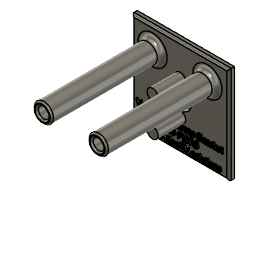
Vekooto Antenna Bracket v1.3 (Autodesk Fusion 360 design; units mm, degrees)
part number: 2026-07-18-22-31-47-243
Autodesk Fusion 360 part; units mm, degrees
note: some values were not read from the file. Chosen so that the rebuilt part matches the saved one: which face or edge a step refers to; the layout of a text; which pieces of a blend or face edit are solid.
(part 1 of 2)
sketch "Sketch1" plane through (0, 0, 0) normal (0, 0, 1) x (1, 0, 0)
  line L0 (22.352, -22.352) -> (-22.352, -22.352)
  line L1 (-22.352, -22.352) -> (-22.352, 22.352)
  line L2 (-22.352, 22.352) -> (22.352, 22.352)
  line L3 (22.352, 22.352) -> (22.352, -22.352)
  line L4 (22.352, -22.352) -> (-22.352, 22.352) construction
  line L5 (-22.352, -22.352) -> (22.352, 22.352) construction
  dimension "d4" = 44.704
  dimension "d5" = 44.704
  constraint horizontal L0
  constraint perpendicular L0 L1
  constraint parallel L0 L2
  constraint parallel L1 L3
  constraint coincident L4 origin
  constraint coincident L5 origin
  measures "d4" distance of L1.end L2.end
  measures "d5" distance of L0.end L1.end
extrude "Extrude1" add sketch "Sketch1" along normal blind 2.54
sketch "Sketch2" plane through (0, 0, 2.54) normal (0, 0, 1) x (1, 0, 0)
  line L0 (22.352, 22.352) -> (-22.352, 22.352)
  line L1 (-22.352, 22.352) -> (-22.352, -22.352)
  line L2 (-22.352, -22.352) -> (22.352, -22.352)
  line L3 (22.352, -22.352) -> (22.352, 22.352)
  circle A0 centre (0, 0) radius 5.08
  dimension "d8" = 10.16
  constraint coincident A0.centre origin
  measures "d8" diameter of A0
extrude "Extrude2" cut sketch "Sketch2" against normal blind 2.54 contours A0
sketch "Sketch3" plane through (0, 0, 2.54) normal (0, 0, 1) x (1, 0, 0)
  circle A0 centre (0, 0) radius 5.08
  line L0 (22.352, 22.352) -> (-22.352, 22.352)
  line L1 (-22.352, 22.352) -> (-22.352, -22.352)
  line L2 (-22.352, -22.352) -> (22.352, -22.352)
  line L3 (22.352, -22.352) -> (22.352, 22.352)
  circle A1 centre (-15.8649, 0) radius 4.445
  dimension "d13" = 8.89
  measures "d13" diameter of A1
extrude "Extrude3" add sketch "Sketch3" along normal blind 50.8 contours A1
move_face "MoveFace1" to x (1, 0, 0) y (0, 1, 0) z (0, 0, 1) at (2.54, 0, 0) 1 faces at (-11.442, -0.4426, 36.4067)
move_face "MoveFace2" to x (1, 0, 0) y (0, 1, 0) z (0, 0, 1) at (2.54, 12.7, 0) 2 faces at (-8.902, 0.4426, 36.4067) (-13.1059, 0.033, 53.34)
sketch "Sketch4" plane through (0, 0, 2.54) normal (0, 0, 1) x (1, 0, 0)
  circle A0 centre (-10.7849, 12.7) radius 4.445
  circle A1 centre (0, 0) radius 5.08
  line L0 (22.352, 22.352) -> (-22.352, 22.352)
  line L1 (-22.352, 22.352) -> (-22.352, -22.352)
  line L2 (-22.352, -22.352) -> (22.352, -22.352)
  line L3 (22.352, -22.352) -> (22.352, 22.352)
  circle A2 centre (11.9328, 13.2113) radius 4.445
  dimension "d18" = 8.89
  measures "d18" diameter of A2
extrude "Extrude4" add sketch "Sketch4" along normal blind 50.8 contours A2
move_face "MoveFace3" to x (1, 0, 0) y (0, 1, 0) z (0, 0, 1) at (0, -0.508, 0) 1 faces at (16.3557, 12.7687, 36.4067)
move_face "MoveFace4" to x (1, 0, 0) y (0, 1, 0) z (0, 0, 1) at (-2.54, 0, 0) 1 faces at (-6.362, 13.1426, 36.4067)
move_face "MoveFace5" to x (1, 0, 0) y (0, 1, 0) z (0, 0, 1) at (0.508, 0, 0) 1 faces at (16.3557, 13.1458, 36.4067)
move_face "MoveFace6" to x (1, 0, 0) y (0, 1, 0) z (0, 0, 1) at (0.508, 0, 0) 1 faces at (-8.902, 13.1426, 36.4067)
sketch "Sketch5" plane through (0, 0, 53.34) normal (0, 0, 1) x (1, 0, 0)
  circle A0 centre (-12.8169, 12.7) radius 4.445
  circle A1 centre (-12.8169, 12.7) radius 2.54
  dimension "d22" = 5.08
  constraint concentric A0 A1
  measures "d22" diameter of A1
sketch "Sketch6" plane through (0, 0, 53.34) normal (0, 0, 1) x (1, 0, 0)
  circle A0 centre (12.4408, 12.7033) radius 4.445
  circle A1 centre (12.4408, 12.7033) radius 2.54
  dimension "d23" = 5.08
  constraint concentric A0 A1
  measures "d23" diameter of A1
extrude "Extrude5" cut sketch "Sketch5" against normal blind 50.8 contours A1
extrude "Extrude6" cut sketch "Sketch6" against normal blind 50.8 contours A1
fillet "Fillet1" radius 2.286 1 edges at (8.2966, 14.3106, 2.54)
fillet "Fillet2" radius 2.286 1 edges at (-16.9611, 14.3074, 2.54)
fillet "Fillet3" radius 0.762 4 edges at (-15.185, 13.6185, 53.34) (-16.9611, 11.0926, 53.34) (10.0726, 13.6218, 53.34) (8.2966, 11.0959, 53.34)
fillet "Fillet4" radius 1.016 4 edges at (0, -22.352, 2.54) (-22.352, 0, 2.54) (0, 22.352, 2.54) (22.352, 0, 2.54)
sketch "Sketch7" plane through (0, 0, 0) normal (0, 0, -1) x (-1, 0, 0)
  circle A0 centre (0, 0) radius 5.08
  line L0 (22.352, 22.352) -> (-22.352, 22.352)
  line L1 (-22.352, 22.352) -> (-22.352, -22.352)
  line L2 (-22.352, -22.352) -> (22.352, -22.352)
  line L3 (22.352, -22.352) -> (22.352, 22.352)
  line L4 (-22.3513, 12.9981) -> (22.3527, 13.0094) construction
  line L5 (22.3527, 13.0094) -> (22.3513, 18.5497) construction
  line L6 (22.3513, 18.5497) -> (-22.3527, 18.5384) construction
  line L7 (-22.3527, 18.5384) -> (-22.3513, 12.9981) construction
  dimension "d36" = 2.54
  dimension "d37" = 0
  text T0 "Vekooto Antenna Bracket v.1.1" font "Arial" height 2.54 align centre top in box 44.704 x 5.5403 at (-22.3513, 12.9981) x (1, 0.000252) y (-0.000252, 1) spacing 1 kerned
  constraint coincident L3
  constraint coincident L1
extrude "Extrude7" cut sketch "Sketch7" against normal blind 0.762 text T0
sketch "Sketch8" plane through (0, 0, 0) normal (0, 0, -1) x (-1, 0, 0)
  line L0 (22.352, 22.352) -> (-22.352, 22.352)
  line L1 (-22.352, 22.352) -> (-22.352, -22.352)
  line L2 (-22.352, -22.352) -> (22.352, -22.352)
  line L3 (22.352, -22.352) -> (22.352, 22.352)
  circle A0 centre (0, 0) radius 5.08
  line L4 (-17.5814, 18.5396) -> (-18.5753, 15.9994)
  line L5 (-18.5753, 15.9994) -> (-18.9201, 15.9993)
  line L6 (-18.9201, 15.9993) -> (-19.9049, 18.5391)
  line L7 (-19.9049, 18.5391) -> (-19.541, 18.5391)
  line L8 (-19.541, 18.5391) -> (-18.8804, 16.6941)
  spline S0 degree 3 poles (-18.8804, 16.6941) (-18.8553, 16.6227) (-18.807, 16.4853) (-18.7664, 16.3455) (-18.7469, 16.2783) knots 0 0 0 0 0.022697 0.043678 0.043678 0.043678 0.043678
  spline S1 degree 3 poles (-18.7469, 16.2783) (-18.7264, 16.3478) (-18.6851, 16.4879) (-18.6353, 16.6251) (-18.6102, 16.6942) knots 0 0 0 0 0.021744 0.043787 0.043787 0.043787 0.043787
  line L9 (-18.6102, 16.6942) -> (-17.9245, 18.5395)
  line L10 (-17.9245, 18.5395) -> (-17.5814, 18.5396)
  line L11 (-15.2281, 16.7297) -> (-15.2279, 16.0002)
  line L12 (-15.2279, 16.0002) -> (-15.5398, 16.0001)
  line L13 (-15.5398, 16.0001) -> (-15.5404, 18.5401)
  line L14 (-15.5404, 18.5401) -> (-15.2286, 18.5402)
  line L15 (-15.2286, 18.5402) -> (-15.2282, 17.0918)
  line L16 (-15.2282, 17.0918) -> (-14.4903, 17.8404)
  line L17 (-14.4903, 17.8404) -> (-14.0866, 17.8405)
  line L18 (-14.0866, 17.8405) -> (-14.7899, 17.1577)
  line L19 (-14.7899, 17.1577) -> (-14.0151, 16.0005)
  line L20 (-14.0151, 16.0005) -> (-14.3997, 16.0004)
  line L21 (-14.3997, 16.0004) -> (-15.0081, 16.9411)
  line L22 (-15.0081, 16.9411) -> (-15.2281, 16.7297)
  spline S2 degree 3 poles (-11.0471, 15.9597) (-11.1683, 15.9686) (-11.403, 15.9857) (-11.5842, 16.1351) (-11.6718, 16.2073) knots 0 0 0 0 0.035478 0.06869 0.06869 0.06869 0.06869
  spline S3 degree 3 poles (-11.6718, 16.2073) (-11.7412, 16.3046) (-11.8927, 16.5171) (-11.9041, 16.7791) (-11.9102, 16.9211) knots 0 0 0 0 0.035119 0.076697 0.076697 0.076697 0.076697
  spline S4 degree 3 poles (-11.9102, 16.9211) (-11.9032, 17.076) (-11.8902, 17.3608) (-11.709, 17.5788) (-11.6263, 17.6783) knots 0 0 0 0 0.045048 0.082857 0.082857 0.082857 0.082857
  spline S5 degree 3 poles (-11.6263, 17.6783) (-11.5415, 17.7379) (-11.368, 17.8601) (-11.1561, 17.8752) (-11.0476, 17.8829) knots 0 0 0 0 0.030474 0.062419 0.062419 0.062419 0.062419
  spline S6 degree 3 poles (-11.0476, 17.8829) (-10.928, 17.8737) (-10.6948, 17.8557) (-10.5149, 17.7069) (-10.4273, 17.6344) knots 0 0 0 0 0.035035 0.068301 0.068301 0.068301 0.068301
  spline S7 degree 3 poles (-10.4273, 17.6344) (-10.3571, 17.5394) (-10.2069, 17.336) (-10.1934, 17.0825) (-10.1863, 16.9475) knots 0 0 0 0 0.034681 0.074234 0.074234 0.074234 0.074234
  spline S8 degree 3 poles (-10.1863, 16.9475) (-10.1883, 16.8403) (-10.192, 16.6476) (-10.2617, 16.4683) (-10.2927, 16.3887) knots 0 0 0 0 0.03184 0.057276 0.057276 0.057276 0.057276
  spline S9 degree 3 poles (-10.2927, 16.3887) (-10.3324, 16.3246) (-10.4119, 16.1959) (-10.539, 16.1137) (-10.6028, 16.0724) knots 0 0 0 0 0.022319 0.044787 0.044787 0.044787 0.044787
  spline S10 degree 3 poles (-10.6028, 16.0724) (-10.6725, 16.0396) (-10.8133, 15.9732) (-10.9687, 15.9642) (-11.0471, 15.9597) knots 0 0 0 0 0.022904 0.046226 0.046226 0.046226 0.046226
  spline S11 degree 3 poles (-8.0879, 15.9604) (-8.2091, 15.9693) (-8.4437, 15.9865) (-8.6249, 16.1358) (-8.7125, 16.208) knots 0 0 0 0 0.035479 0.06869 0.06869 0.06869 0.06869
  spline S12 degree 3 poles (-8.7125, 16.208) (-8.7819, 16.3054) (-8.9334, 16.5179) (-8.9448, 16.7798) (-8.9509, 16.9218) knots 0 0 0 0 0.035119 0.076697 0.076697 0.076697 0.076697
  spline S13 degree 3 poles (-8.9509, 16.9218) (-8.9439, 17.0767) (-8.9309, 17.3616) (-8.7497, 17.5796) (-8.667, 17.679) knots 0 0 0 0 0.045048 0.082857 0.082857 0.082857 0.082857
  spline S14 degree 3 poles (-8.667, 17.679) (-8.5823, 17.7387) (-8.4087, 17.8608) (-8.1968, 17.8759) (-8.0883, 17.8836) knots 0 0 0 0 0.030474 0.062419 0.062419 0.062419 0.062419
  spline S15 degree 3 poles (-8.0883, 17.8836) (-7.9687, 17.8744) (-7.7356, 17.8565) (-7.5556, 17.7076) (-7.468, 17.6352) knots 0 0 0 0 0.035035 0.068301 0.068301 0.068301 0.068301
  spline S16 degree 3 poles (-7.468, 17.6352) (-7.3978, 17.5401) (-7.2476, 17.3367) (-7.2342, 17.0833) (-7.227, 16.9482) knots 0 0 0 0 0.034681 0.074234 0.074234 0.074234 0.074234
  spline S17 degree 3 poles (-7.227, 16.9482) (-7.229, 16.8411) (-7.2327, 16.6483) (-7.3025, 16.4691) (-7.3334, 16.3895) knots 0 0 0 0 0.03184 0.057276 0.057276 0.057276 0.057276
  spline S18 degree 3 poles (-7.3334, 16.3895) (-7.3731, 16.3253) (-7.4526, 16.1966) (-7.5797, 16.1144) (-7.6435, 16.0732) knots 0 0 0 0 0.022319 0.044787 0.044787 0.044787 0.044787
  spline S19 degree 3 poles (-7.6435, 16.0732) (-7.7132, 16.0403) (-7.854, 15.974) (-8.0094, 15.965) (-8.0879, 15.9604) knots 0 0 0 0 0.022904 0.046226 0.046226 0.046226 0.046226
  line L23 (-3.3928, 17.0081) -> (-3.3925, 16.0032)
  line L24 (-3.3925, 16.0032) -> (-3.7044, 16.0031)
  line L25 (-3.7044, 16.0031) -> (-3.7048, 17.8432)
  line L26 (-3.7048, 17.8432) -> (-3.4242, 17.8432)
  line L27 (-3.4242, 17.8432) -> (-3.4241, 17.5816)
  spline S20 degree 3 poles (-3.4241, 17.5816) (-3.3481, 17.67) (-3.1939, 17.8496) (-2.9582, 17.873) (-2.8385, 17.885) knots 0 0 0 0 0.03363 0.068256 0.068256 0.068256 0.068256
  spline S21 degree 3 poles (-2.8385, 17.885) (-2.7848, 17.8827) (-2.6798, 17.8784) (-2.581, 17.8427) (-2.5327, 17.8253) knots 0 0 0 0 0.016031 0.031322 0.031322 0.031322 0.031322
  spline S22 degree 3 poles (-2.5327, 17.8253) (-2.49, 17.8049) (-2.4097, 17.7667) (-2.3513, 17.6998) (-2.3239, 17.6685) knots 0 0 0 0 0.014014 0.026358 0.026358 0.026358 0.026358
  spline S23 degree 3 poles (-2.3239, 17.6685) (-2.3024, 17.6339) (-2.2578, 17.5623) (-2.2374, 17.4804) (-2.2268, 17.4381) knots 0 0 0 0 0.012138 0.02514 0.02514 0.02514 0.02514
  spline S24 degree 3 poles (-2.2268, 17.4381) (-2.2218, 17.3984) (-2.2091, 17.2978) (-2.2093, 17.1964) (-2.2094, 17.1349) knots 0 0 0 0 0.011982 0.030396 0.030396 0.030396 0.030396
  line L28 (-2.2094, 17.1349) -> (-2.2091, 16.0035)
  line L29 (-2.2091, 16.0035) -> (-2.521, 16.0034)
  line L30 (-2.521, 16.0034) -> (-2.5213, 17.1227)
  spline S25 degree 3 poles (-2.5213, 17.1227) (-2.5216, 17.1786) (-2.5221, 17.2752) (-2.5472, 17.3684) (-2.5577, 17.4077) knots 0 0 0 0 0.016679 0.028836 0.028836 0.028836 0.028836
  spline S26 degree 3 poles (-2.5577, 17.4077) (-2.5725, 17.4377) (-2.6026, 17.499) (-2.6584, 17.5384) (-2.6869, 17.5584) knots 0 0 0 0 0.009876 0.020131 0.020131 0.020131 0.020131
  spline S27 degree 3 poles (-2.6869, 17.5584) (-2.7198, 17.5748) (-2.7882, 17.6089) (-2.8647, 17.6127) (-2.9043, 17.6147) knots 0 0 0 0 0.01092 0.022678 0.022678 0.022678 0.022678
  spline S28 degree 3 poles (-2.9043, 17.6147) (-2.9682, 17.6096) (-3.0947, 17.5995) (-3.1974, 17.525) (-3.2482, 17.4881) knots 0 0 0 0 0.018828 0.037284 0.037284 0.037284 0.037284
  spline S29 degree 3 poles (-3.2482, 17.4881) (-3.2901, 17.429) (-3.3908, 17.2868) (-3.392, 17.1109) (-3.3928, 17.0081) knots 0 0 0 0 0.021294 0.051185 0.051185 0.051185 0.051185
  spline S30 degree 3 poles (0.0293, 16.2189) (0.0837, 16.2221) (0.1888, 16.2284) (0.2787, 16.2828) (0.3221, 16.3091) knots 0 0 0 0 0.016056 0.031049 0.031049 0.031049 0.031049
  spline S31 degree 3 poles (0.3221, 16.3091) (0.3613, 16.3461) (0.4471, 16.427) (0.4907, 16.537) (0.5144, 16.5967) knots 0 0 0 0 0.015968 0.034972 0.034972 0.034972 0.034972
  line L31 (0.5144, 16.5967) -> (0.8366, 16.557)
  spline S32 degree 3 poles (0.8366, 16.557) (0.8071, 16.469) (0.7498, 16.2989) (0.618, 16.1773) (0.5543, 16.1185) knots 0 0 0 0 0.027335 0.052897 0.052897 0.052897 0.052897
  spline S33 degree 3 poles (0.5543, 16.1185) (0.4781, 16.0731) (0.3162, 15.9766) (0.1275, 15.9674) (0.0277, 15.9625) knots 0 0 0 0 0.026229 0.055682 0.055682 0.055682 0.055682
  spline S34 degree 3 poles (0.0277, 15.9625) (-0.0979, 15.9708) (-0.3381, 15.9866) (-0.5239, 16.1385) (-0.6126, 16.2109) knots 0 0 0 0 0.03672 0.070219 0.070219 0.070219 0.070219
  spline S35 degree 3 poles (-0.6126, 16.2109) (-0.6815, 16.307) (-0.8303, 16.5146) (-0.8427, 16.7707) (-0.8493, 16.9083) knots 0 0 0 0 0.034736 0.075044 0.075044 0.075044 0.075044
  spline S36 degree 3 poles (-0.8493, 16.9083) (-0.8428, 17.0504) (-0.8308, 17.3142) (-0.6799, 17.5297) (-0.6103, 17.6291) knots 0 0 0 0 0.041667 0.077342 0.077342 0.077342 0.077342
  spline S37 degree 3 poles (-0.6103, 17.6291) (-0.5233, 17.7039) (-0.345, 17.8571) (-0.1103, 17.876) (0.0099, 17.8857) knots 0 0 0 0 0.033526 0.068681 0.068681 0.068681 0.068681
  spline S38 degree 3 poles (0.0099, 17.8857) (0.1264, 17.8761) (0.3548, 17.8574) (0.528, 17.7078) (0.6129, 17.6346) knots 0 0 0 0 0.034109 0.066844 0.066844 0.066844 0.066844
  spline S39 degree 3 poles (0.6129, 17.6346) (0.681, 17.5372) (0.8288, 17.3259) (0.8406, 17.0672) (0.847, 16.9277) knots 0 0 0 0 0.034955 0.075831 0.075831 0.075831 0.075831
  spline S40 degree 3 poles (0.847, 16.9277) (0.8468, 16.9162) (0.8466, 16.8885) (0.8457, 16.8608) (0.8452, 16.8446) knots 0 0 0 0 0.003465 0.008319 0.008319 0.008319 0.008319
  line L32 (0.8452, 16.8446) -> (-0.527, 16.8442)
  spline S41 degree 3 poles (-0.527, 16.8442) (-0.5179, 16.7519) (-0.5013, 16.5814) (-0.4012, 16.4432) (-0.3553, 16.3799) knots 0 0 0 0 0.02726 0.050297 0.050297 0.050297 0.050297
  spline S42 degree 3 poles (-0.3553, 16.3799) (-0.3004, 16.333) (-0.1895, 16.2381) (-0.0441, 16.2254) (0.0293, 16.2189) knots 0 0 0 0 0.021124 0.042642 0.042642 0.042642 0.042642
  line L33 (3.5134, 17.0099) -> (3.5137, 16.0049)
  line L34 (3.5137, 16.0049) -> (3.2018, 16.0049)
  line L35 (3.2018, 16.0049) -> (3.2013, 17.8449)
  line L36 (3.2013, 17.8449) -> (3.482, 17.845)
  line L37 (3.482, 17.845) -> (3.4821, 17.5833)
  spline S43 degree 3 poles (3.4821, 17.5833) (3.558, 17.6718) (3.7122, 17.8513) (3.948, 17.8748) (4.0676, 17.8867) knots 0 0 0 0 0.03363 0.068256 0.068256 0.068256 0.068256
  spline S44 degree 3 poles (4.0676, 17.8867) (4.1214, 17.8845) (4.2264, 17.8801) (4.3252, 17.8444) (4.3734, 17.827) knots 0 0 0 0 0.016031 0.031322 0.031322 0.031322 0.031322
  spline S45 degree 3 poles (4.3734, 17.827) (4.4162, 17.8067) (4.4965, 17.7685) (4.5549, 17.7016) (4.5823, 17.6702) knots 0 0 0 0 0.014014 0.026358 0.026358 0.026358 0.026358
  spline S46 degree 3 poles (4.5823, 17.6702) (4.6038, 17.6357) (4.6484, 17.5641) (4.6688, 17.4822) (4.6793, 17.4398) knots 0 0 0 0 0.012138 0.02514 0.02514 0.02514 0.02514
  spline S47 degree 3 poles (4.6793, 17.4398) (4.6844, 17.4002) (4.6971, 17.2996) (4.6969, 17.1981) (4.6968, 17.1366) knots 0 0 0 0 0.011982 0.030396 0.030396 0.030396 0.030396
  line L38 (4.6968, 17.1366) -> (4.697, 16.0052)
  line L39 (4.697, 16.0052) -> (4.3852, 16.0052)
  line L40 (4.3852, 16.0052) -> (4.3849, 17.1244)
  spline S48 degree 3 poles (4.3849, 17.1244) (4.3846, 17.1803) (4.384, 17.277) (4.359, 17.3701) (4.3484, 17.4094) knots 0 0 0 0 0.016679 0.028836 0.028836 0.028836 0.028836
  spline S49 degree 3 poles (4.3484, 17.4094) (4.3337, 17.4395) (4.3036, 17.5007) (4.2478, 17.5401) (4.2193, 17.5601) knots 0 0 0 0 0.009876 0.02013 0.02013 0.02013 0.02013
  spline S50 degree 3 poles (4.2193, 17.5601) (4.1864, 17.5765) (4.1179, 17.6106) (4.0415, 17.6144) (4.0019, 17.6164) knots 0 0 0 0 0.01092 0.022678 0.022678 0.022678 0.022678
  spline S51 degree 3 poles (4.0019, 17.6164) (3.938, 17.6113) (3.8114, 17.6013) (3.7088, 17.5267) (3.658, 17.4898) knots 0 0 0 0 0.018828 0.037284 0.037284 0.037284 0.037284
  spline S52 degree 3 poles (3.658, 17.4898) (3.6161, 17.4307) (3.5154, 17.2886) (3.5141, 17.1126) (3.5134, 17.0099) knots 0 0 0 0 0.021294 0.051185 0.051185 0.051185 0.051185
  line L41 (6.764, 16.0058) -> (6.4383, 16.0057)
  spline S53 degree 3 poles (6.4383, 16.0057) (6.4235, 16.0403) (6.3923, 16.1131) (6.3815, 16.1915) (6.3759, 16.2326) knots 0 0 0 0 0.011255 0.023633 0.023633 0.023633 0.023633
  spline S54 degree 3 poles (6.3759, 16.2326) (6.3209, 16.188) (6.2183, 16.1048) (6.0982, 16.05) (6.0424, 16.0246) knots 0 0 0 0 0.021138 0.039444 0.039444 0.039444 0.039444
  spline S55 degree 3 poles (6.0424, 16.0246) (5.9875, 16.0069) (5.8757, 15.9709) (5.7582, 15.9663) (5.6985, 15.9639) knots 0 0 0 0 0.017222 0.035068 0.035068 0.035068 0.035068
  spline S56 degree 3 poles (5.6985, 15.9639) (5.6062, 15.9676) (5.4365, 15.9743) (5.2963, 16.0688) (5.2324, 16.1119) knots 0 0 0 0 0.027067 0.049766 0.049766 0.049766 0.049766
  spline S57 degree 3 poles (5.2324, 16.1119) (5.1849, 16.1652) (5.0886, 16.2732) (5.0759, 16.4174) (5.0694, 16.4905) knots 0 0 0 0 0.020829 0.042207 0.042207 0.042207 0.042207
  spline S58 degree 3 poles (5.0694, 16.4905) (5.0718, 16.5342) (5.0765, 16.6205) (5.1129, 16.6988) (5.1309, 16.7374) knots 0 0 0 0 0.013021 0.025653 0.025653 0.025653 0.025653
  spline S59 degree 3 poles (5.1309, 16.7374) (5.1527, 16.7726) (5.1957, 16.842) (5.2602, 16.8921) (5.292, 16.9167) knots 0 0 0 0 0.012324 0.024281 0.024281 0.024281 0.024281
  spline S60 degree 3 poles (5.292, 16.9167) (5.3266, 16.938) (5.3971, 16.9813) (5.4761, 17.0063) (5.5163, 17.019) knots 0 0 0 0 0.01214 0.024739 0.024739 0.024739 0.024739
  spline S61 degree 3 poles (5.5163, 17.019) (5.5546, 17.0275) (5.6462, 17.0477) (5.7393, 17.0592) (5.7935, 17.0659) knots 0 0 0 0 0.011766 0.028127 0.028127 0.028127 0.028127
  spline S62 degree 3 poles (5.7935, 17.0659) (5.9034, 17.0792) (6.0915, 17.102) (6.2739, 17.1525) (6.3496, 17.1734) knots 0 0 0 0 0.033159 0.056713 0.056713 0.056713 0.056713
  spline S63 degree 3 poles (6.3496, 17.1734) (6.3501, 17.1909) (6.3509, 17.218) (6.3512, 17.2452) (6.3514, 17.2549) knots 0 0 0 0 0.005243 0.008145 0.008145 0.008145 0.008145
  spline S64 degree 3 poles (6.3514, 17.2549) (6.3501, 17.3112) (6.3479, 17.4106) (6.2886, 17.4893) (6.2629, 17.5234) knots 0 0 0 0 0.016393 0.028904 0.028904 0.028904 0.028904
  spline S65 degree 3 poles (6.2629, 17.5234) (6.2148, 17.5541) (6.107, 17.6228) (5.9787, 17.6268) (5.9077, 17.629) knots 0 0 0 0 0.016839 0.037669 0.037669 0.037669 0.037669
  spline S66 degree 3 poles (5.9077, 17.629) (5.8426, 17.628) (5.7281, 17.6262) (5.6266, 17.5742) (5.5829, 17.5518) knots 0 0 0 0 0.01922 0.03378 0.03378 0.03378 0.03378
  spline S67 degree 3 poles (5.5829, 17.5518) (5.5495, 17.518) (5.4738, 17.4413) (5.4443, 17.3371) (5.4279, 17.2789) knots 0 0 0 0 0.014041 0.031838 0.031838 0.031838 0.031838
  line L42 (5.4279, 17.2789) -> (5.1229, 17.3204)
  spline S68 degree 3 poles (5.1229, 17.3204) (5.1378, 17.3809) (5.1656, 17.4942) (5.2298, 17.5914) (5.2597, 17.6366) knots 0 0 0 0 0.01853 0.034684 0.034684 0.034684 0.034684
  spline S69 degree 3 poles (5.2597, 17.6366) (5.2966, 17.675) (5.3749, 17.7565) (5.4797, 17.7994) (5.5352, 17.8221) knots 0 0 0 0 0.01579 0.033533 0.033533 0.033533 0.033533
  spline S70 degree 3 poles (5.5352, 17.8221) (5.5995, 17.841) (5.7358, 17.8811) (5.8778, 17.8851) (5.9527, 17.8872) knots 0 0 0 0 0.02005 0.042416 0.042416 0.042416 0.042416
  spline S71 degree 3 poles (5.9527, 17.8872) (6.0244, 17.886) (6.1546, 17.8838) (6.2795, 17.8479) (6.3356, 17.8318) knots 0 0 0 0 0.021399 0.038838 0.038838 0.038838 0.038838
  spline S72 degree 3 poles (6.3356, 17.8318) (6.3801, 17.8138) (6.4612, 17.7808) (6.5239, 17.7199) (6.5522, 17.6924) knots 0 0 0 0 0.014228 0.025974 0.025974 0.025974 0.025974
  spline S73 degree 3 poles (6.5522, 17.6924) (6.5738, 17.6616) (6.6191, 17.5969) (6.6389, 17.5203) (6.6493, 17.4802) knots 0 0 0 0 0.011185 0.023506 0.023506 0.023506 0.023506
  spline S74 degree 3 poles (6.6493, 17.4802) (6.6538, 17.443) (6.6654, 17.3475) (6.6651, 17.2513) (6.665, 17.1926) knots 0 0 0 0 0.011236 0.028827 0.028827 0.028827 0.028827
  line L43 (6.665, 17.1926) -> (6.6651, 16.7767)
  spline S75 degree 3 poles (6.6651, 16.7767) (6.6644, 16.6583) (6.6633, 16.4746) (6.6794, 16.2917) (6.6851, 16.2266) knots 0 0 0 0 0.0355 0.055071 0.055071 0.055071 0.055071
  spline S76 degree 3 poles (6.6851, 16.2266) (6.6935, 16.1885) (6.7104, 16.1115) (6.746, 16.0412) (6.764, 16.0058) knots 0 0 0 0 0.011667 0.02354 0.02354 0.02354 0.02354
  line L44 (10.8094, 16.9701) -> (10.8097, 16.0068)
  line L45 (10.8097, 16.0068) -> (10.4978, 16.0067)
  line L46 (10.4978, 16.0067) -> (10.4973, 17.8467)
  line L47 (10.4973, 17.8467) -> (10.778, 17.8468)
  line L48 (10.778, 17.8468) -> (10.7781, 17.5678)
  spline S77 degree 3 poles (10.7781, 17.5678) (10.8093, 17.6245) (10.8625, 17.7209) (10.9432, 17.7954) (10.9764, 17.8261) knots 0 0 0 0 0.01925 0.032742 0.032742 0.032742 0.032742
  spline S78 degree 3 poles (10.9764, 17.8261) (11.0074, 17.8443) (11.0693, 17.8806) (11.1408, 17.8858) (11.1765, 17.8885) knots 0 0 0 0 0.010635 0.021211 0.021211 0.021211 0.021211
  spline S79 degree 3 poles (11.1765, 17.8885) (11.2305, 17.8835) (11.3444, 17.873) (11.4445, 17.8173) (11.4971, 17.7881) knots 0 0 0 0 0.016094 0.033922 0.033922 0.033922 0.033922
  line L49 (11.4971, 17.7881) -> (11.3897, 17.4987)
  spline S80 degree 3 poles (11.3897, 17.4987) (11.3524, 17.5184) (11.2806, 17.5563) (11.1998, 17.563) (11.161, 17.5662) knots 0 0 0 0 0.012508 0.024067 0.024067 0.024067 0.024067
  spline S81 degree 3 poles (11.161, 17.5662) (11.1278, 17.5636) (11.0614, 17.5585) (11.0054, 17.5226) (10.9774, 17.5047) knots 0 0 0 0 0.009824 0.019638 0.019638 0.019638 0.019638
  spline S82 degree 3 poles (10.9774, 17.5047) (10.952, 17.4816) (10.8997, 17.4341) (10.8744, 17.368) (10.8613, 17.334) knots 0 0 0 0 0.010126 0.020898 0.020898 0.020898 0.020898
  spline S83 degree 3 poles (10.8613, 17.334) (10.8462, 17.2762) (10.8149, 17.157) (10.8113, 17.0337) (10.8094, 16.9701) knots 0 0 0 0 0.017844 0.03686 0.03686 0.03686 0.03686
  spline S84 degree 3 poles (14.3944, 16.2225) (14.4525, 16.2267) (14.5657, 16.2349) (14.6567, 16.3024) (14.701, 16.3352) knots 0 0 0 0 0.017083 0.033278 0.033278 0.033278 0.033278
  spline S85 degree 3 poles (14.701, 16.3352) (14.7386, 16.3809) (14.8216, 16.4819) (14.8444, 16.6111) (14.8569, 16.6818) knots 0 0 0 0 0.017473 0.038572 0.038572 0.038572 0.038572
  line L50 (14.8569, 16.6818) -> (15.1635, 16.642)
  spline S86 degree 3 poles (15.1635, 16.642) (15.1419, 16.5435) (15.1004, 16.3546) (14.9692, 16.2132) (14.9064, 16.1455) knots 0 0 0 0 0.029645 0.056823 0.056823 0.056823 0.056823
  spline S87 degree 3 poles (14.9064, 16.1455) (14.8322, 16.0932) (14.6798, 15.9858) (14.4935, 15.9728) (14.3979, 15.9661) knots 0 0 0 0 0.0267 0.054846 0.054846 0.054846 0.054846
  spline S88 degree 3 poles (14.3979, 15.9661) (14.2795, 15.975) (14.0501, 15.9921) (13.8752, 16.1409) (13.7906, 16.2128) knots 0 0 0 0 0.034622 0.067083 0.067083 0.067083 0.067083
  spline S89 degree 3 poles (13.7906, 16.2128) (13.7237, 16.3097) (13.5774, 16.5217) (13.5667, 16.7802) (13.5608, 16.9206) knots 0 0 0 0 0.034624 0.075764 0.075764 0.075764 0.075764
  spline S90 degree 3 poles (13.5608, 16.9206) (13.564, 17.0147) (13.5701, 17.1937) (13.6307, 17.3622) (13.6594, 17.4421) knots 0 0 0 0 0.028047 0.053368 0.053368 0.053368 0.053368
  spline S91 degree 3 poles (13.6594, 17.4421) (13.6961, 17.5116) (13.7683, 17.6486) (13.8967, 17.7349) (13.96, 17.7774) knots 0 0 0 0 0.023185 0.045661 0.045661 0.045661 0.045661
  spline S92 degree 3 poles (13.96, 17.7774) (14.029, 17.81) (14.1681, 17.8757) (14.3218, 17.8848) (14.3992, 17.8893) knots 0 0 0 0 0.022679 0.045697 0.045697 0.045697 0.045697
  spline S93 degree 3 poles (14.3992, 17.8893) (14.4925, 17.8845) (14.6692, 17.8756) (14.8189, 17.782) (14.8895, 17.7378) knots 0 0 0 0 0.027507 0.052083 0.052083 0.052083 0.052083
  spline S94 degree 3 poles (14.8895, 17.7378) (14.9477, 17.6802) (15.0692, 17.5598) (15.1117, 17.3938) (15.1339, 17.3073) knots 0 0 0 0 0.024104 0.050333 0.050333 0.050333 0.050333
  line L51 (15.1339, 17.3073) -> (14.8307, 17.2605)
  spline S95 degree 3 poles (14.8307, 17.2605) (14.815, 17.317) (14.7858, 17.4224) (14.7117, 17.5024) (14.6773, 17.5394) knots 0 0 0 0 0.017316 0.032245 0.032245 0.032245 0.032245
  spline S96 degree 3 poles (14.6773, 17.5394) (14.6382, 17.5666) (14.5583, 17.6224) (14.461, 17.6293) (14.4113, 17.6329) knots 0 0 0 0 0.014031 0.028664 0.028664 0.028664 0.028664
  spline S97 degree 3 poles (14.4113, 17.6329) (14.3369, 17.6262) (14.19, 17.6131) (14.0818, 17.5131) (14.0285, 17.4638) knots 0 0 0 0 0.021768 0.042919 0.042919 0.042919 0.042919
  spline S98 degree 3 poles (14.0285, 17.4638) (13.9857, 17.3929) (13.8873, 17.2296) (13.8835, 17.0378) (13.8813, 16.9293) knots 0 0 0 0 0.024447 0.056302 0.056302 0.056302 0.056302
  spline S99 degree 3 poles (13.8813, 16.9293) (13.8832, 16.8197) (13.8864, 16.6273) (13.9823, 16.4617) (14.0236, 16.3905) knots 0 0 0 0 0.032206 0.056538 0.056538 0.056538 0.056538
  spline S100 degree 3 poles (14.0236, 16.3905) (14.075, 16.3415) (14.1789, 16.2424) (14.322, 16.2292) (14.3944, 16.2225) knots 0 0 0 0 0.020663 0.04179 0.04179 0.04179 0.04179
  spline S101 degree 3 poles (17.9791, 16.2234) (18.0335, 16.2266) (18.1386, 16.2329) (18.2285, 16.2873) (18.2719, 16.3136) knots 0 0 0 0 0.016055 0.031048 0.031048 0.031048 0.031048
  spline S102 degree 3 poles (18.2719, 16.3136) (18.3111, 16.3506) (18.3968, 16.4316) (18.4405, 16.5415) (18.4642, 16.6013) knots 0 0 0 0 0.015968 0.034972 0.034972 0.034972 0.034972
  line L52 (18.4642, 16.6013) -> (18.7864, 16.5615)
  spline S103 degree 3 poles (18.7864, 16.5615) (18.7569, 16.4736) (18.6996, 16.3034) (18.5678, 16.1818) (18.5041, 16.1231) knots 0 0 0 0 0.027335 0.052897 0.052897 0.052897 0.052897
  spline S104 degree 3 poles (18.5041, 16.1231) (18.4279, 16.0776) (18.266, 15.9811) (18.0773, 15.9719) (17.9775, 15.967) knots 0 0 0 0 0.026228 0.055682 0.055682 0.055682 0.055682
  spline S105 degree 3 poles (17.9775, 15.967) (17.8519, 15.9753) (17.6117, 15.9911) (17.4259, 16.143) (17.3372, 16.2155) knots 0 0 0 0 0.036719 0.070219 0.070219 0.070219 0.070219
  spline S106 degree 3 poles (17.3372, 16.2155) (17.2683, 16.3115) (17.1194, 16.5191) (17.1071, 16.7752) (17.1005, 16.9128) knots 0 0 0 0 0.034736 0.075044 0.075044 0.075044 0.075044
  spline S107 degree 3 poles (17.1005, 16.9128) (17.107, 17.0549) (17.119, 17.3188) (17.2699, 17.5342) (17.3395, 17.6336) knots 0 0 0 0 0.041667 0.077342 0.077342 0.077342 0.077342
  spline S108 degree 3 poles (17.3395, 17.6336) (17.4265, 17.7084) (17.6048, 17.8616) (17.8395, 17.8805) (17.9597, 17.8902) knots 0 0 0 0 0.033526 0.068681 0.068681 0.068681 0.068681
  spline S109 degree 3 poles (17.9597, 17.8902) (18.0762, 17.8806) (18.3046, 17.8619) (18.4778, 17.7124) (18.5627, 17.6391) knots 0 0 0 0 0.034109 0.066844 0.066844 0.066844 0.066844
  spline S110 degree 3 poles (18.5627, 17.6391) (18.6308, 17.5417) (18.7786, 17.3304) (18.7904, 17.0717) (18.7968, 16.9323) knots 0 0 0 0 0.034955 0.075831 0.075831 0.075831 0.075831
  spline S111 degree 3 poles (18.7968, 16.9323) (18.7966, 16.9207) (18.7964, 16.893) (18.7955, 16.8653) (18.795, 16.8491) knots 0 0 0 0 0.003465 0.008319 0.008319 0.008319 0.008319
  line L53 (18.795, 16.8491) -> (17.4228, 16.8488)
  spline S112 degree 3 poles (17.4228, 16.8488) (17.4318, 16.7564) (17.4485, 16.5859) (17.5486, 16.4477) (17.5945, 16.3845) knots 0 0 0 0 0.027261 0.050297 0.050297 0.050297 0.050297
  spline S113 degree 3 poles (17.5945, 16.3845) (17.6494, 16.3375) (17.7603, 16.2426) (17.9057, 16.2299) (17.9791, 16.2234) knots 0 0 0 0 0.021125 0.042643 0.042643 0.042643 0.042643
  line L54 (-1.9764, 13.8794) -> (-2.6725, 12.0392)
  line L55 (-2.6725, 12.0392) -> (-2.9636, 12.0391)
  line L56 (-2.9636, 12.0391) -> (-3.664, 13.879)
  line L57 (-3.664, 13.879) -> (-3.3348, 13.879)
  line L58 (-3.3348, 13.879) -> (-2.9395, 12.7772)
  spline S114 degree 3 poles (-2.9395, 12.7772) (-2.9184, 12.7167) (-2.8757, 12.5942) (-2.8398, 12.4696) (-2.8216, 12.4065) knots 0 0 0 0 0.019204 0.038911 0.038911 0.038911 0.038911
  spline S115 degree 3 poles (-2.8216, 12.4065) (-2.8054, 12.46) (-2.7699, 12.5777) (-2.7282, 12.6934) (-2.7056, 12.7565) knots 0 0 0 0 0.016783 0.036879 0.036879 0.036879 0.036879
  line L59 (-2.7056, 12.7565) -> (-2.297, 13.8793)
  line L60 (-2.297, 13.8793) -> (-1.9764, 13.8794)
  line L61 (-0.0915, 14.5902) -> (0.1095, 14.5903)
  line L62 (0.1095, 14.5903) -> (0.1101, 12.0399)
  line L63 (0.1101, 12.0399) -> (-0.2018, 12.0398)
  line L64 (-0.2018, 12.0398) -> (-0.2023, 14.0271)
  spline S116 degree 3 poles (-0.2023, 14.0271) (-0.2448, 13.9901) (-0.3369, 13.9099) (-0.4414, 13.8464) (-0.4976, 13.8122) knots 0 0 0 0 0.016876 0.036586 0.036586 0.036586 0.036586
  spline S117 degree 3 poles (-0.4976, 13.8122) (-0.5548, 13.7794) (-0.6608, 13.7187) (-0.7738, 13.6723) (-0.8259, 13.651) knots 0 0 0 0 0.01973 0.036608 0.036608 0.036608 0.036608
  line L65 (-0.8259, 13.651) -> (-0.826, 13.9524)
  spline S118 degree 3 poles (-0.826, 13.9524) (-0.7424, 13.9949) (-0.5791, 14.0778) (-0.4377, 14.1939) (-0.3687, 14.2506) knots 0 0 0 0 0.028036 0.054737 0.054737 0.054737 0.054737
  spline S119 degree 3 poles (-0.3687, 14.2506) (-0.3097, 14.3055) (-0.2017, 14.4062) (-0.126, 14.5327) (-0.0915, 14.5902) knots 0 0 0 0 0.024015 0.04403 0.04403 0.04403 0.04403
  line L66 (1.4389, 12.3954) -> (1.439, 12.0402)
  line L67 (1.439, 12.0402) -> (1.0838, 12.0401)
  line L68 (1.0838, 12.0401) -> (1.0837, 12.3953)
  line L69 (1.0837, 12.3953) -> (1.4389, 12.3954)
  line L70 (-1.5204, 12.3947) -> (-1.5203, 12.0395)
  line L71 (-1.5203, 12.0395) -> (-1.8755, 12.0394)
  line L72 (-1.8755, 12.0394) -> (-1.8756, 12.3946)
  line L73 (-1.8756, 12.3946) -> (-1.5204, 12.3947)
  spline S120 degree 3 poles (19.6156, 16.2983) (19.6304, 16.2918) (19.6643, 16.2769) (19.7014, 16.2762) (19.7221, 16.2758) knots 0 0 0 0 0.004831 0.010986 0.010986 0.010986 0.010986
  spline S121 degree 3 poles (19.7221, 16.2758) (19.7422, 16.2766) (19.788, 16.2782) (19.8335, 16.2845) (19.859, 16.288) knots 0 0 0 0 0.006028 0.013749 0.013749 0.013749 0.013749
  line L74 (19.859, 16.288) -> (19.9041, 16.0125)
  spline S122 degree 3 poles (19.9041, 16.0125) (19.8627, 16.0044) (19.7848, 15.9893) (19.7055, 15.9862) (19.6685, 15.9847) knots 0 0 0 0 0.012647 0.023757 0.023757 0.023757 0.023757
  spline S123 degree 3 poles (19.6685, 15.9847) (19.6175, 15.9857) (19.5261, 15.9874) (19.4422, 16.0228) (19.4051, 16.0384) knots 0 0 0 0 0.015133 0.027094 0.027094 0.027094 0.027094
  spline S124 degree 3 poles (19.4051, 16.0384) (19.3765, 16.0572) (19.321, 16.0936) (19.2889, 16.1515) (19.2734, 16.1796) knots 0 0 0 0 0.010107 0.019568 0.019568 0.019568 0.019568
  spline S125 degree 3 poles (19.2734, 16.1796) (19.2624, 16.2246) (19.2331, 16.3453) (19.2344, 16.4698) (19.2352, 16.5477) knots 0 0 0 0 0.013877 0.037135 0.037135 0.037135 0.037135
  line L75 (19.2352, 16.5477) -> (19.2349, 17.6064)
  line L76 (19.2349, 17.6064) -> (19.0062, 17.6063)
  line L77 (19.0062, 17.6063) -> (19.0062, 17.8489)
  line L78 (19.0062, 17.8489) -> (19.2349, 17.8489)
  line L79 (19.2349, 17.8489) -> (19.2347, 18.3046)
  line L80 (19.2347, 18.3046) -> (19.5448, 18.4918)
  line L81 (19.5448, 18.4918) -> (19.545, 17.849)
  line L82 (19.545, 17.849) -> (19.8586, 17.8491)
  line L83 (19.8586, 17.8491) -> (19.8587, 17.6065)
  line L84 (19.8587, 17.6065) -> (19.5451, 17.6064)
  line L85 (19.5451, 17.6064) -> (19.5453, 16.5305)
  spline S126 degree 3 poles (19.5453, 16.5305) (19.5449, 16.4937) (19.5442, 16.4358) (19.5571, 16.3795) (19.5618, 16.359) knots 0 0 0 0 0.010966 0.017282 0.017282 0.017282 0.017282
  spline S127 degree 3 poles (19.5618, 16.359) (19.5683, 16.3469) (19.5813, 16.3223) (19.604, 16.3064) (19.6156, 16.2983) knots 0 0 0 0 0.00405 0.008204 0.008204 0.008204 0.008204
  line L86 (15.7439, 16.7374) -> (15.7441, 16.008)
  line L87 (15.7441, 16.008) -> (15.4323, 16.0079)
  line L88 (15.4323, 16.0079) -> (15.4316, 18.5479)
  line L89 (15.4316, 18.5479) -> (15.7435, 18.548)
  line L90 (15.7435, 18.548) -> (15.7439, 17.0996)
  line L91 (15.7439, 17.0996) -> (16.4818, 17.8482)
  line L92 (16.4818, 17.8482) -> (16.8855, 17.8483)
  line L93 (16.8855, 17.8483) -> (16.1822, 17.1655)
  line L94 (16.1822, 17.1655) -> (16.957, 16.0083)
  line L95 (16.957, 16.0083) -> (16.5723, 16.0082)
  line L96 (16.5723, 16.0082) -> (15.9639, 16.9489)
  line L97 (15.9639, 16.9489) -> (15.7439, 16.7374)
  line L98 (13.2717, 16.0074) -> (12.946, 16.0073)
  spline S128 degree 3 poles (12.946, 16.0073) (12.9311, 16.042) (12.9, 16.1147) (12.8892, 16.1932) (12.8835, 16.2343) knots 0 0 0 0 0.011255 0.023633 0.023633 0.023633 0.023633
  spline S129 degree 3 poles (12.8835, 16.2343) (12.8286, 16.1897) (12.726, 16.1064) (12.6058, 16.0517) (12.5501, 16.0263) knots 0 0 0 0 0.021138 0.039444 0.039444 0.039444 0.039444
  spline S130 degree 3 poles (12.5501, 16.0263) (12.4951, 16.0086) (12.3833, 15.9725) (12.2659, 15.9679) (12.2062, 15.9655) knots 0 0 0 0 0.017222 0.035068 0.035068 0.035068 0.035068
  spline S131 degree 3 poles (12.2062, 15.9655) (12.1139, 15.9692) (11.9442, 15.976) (11.804, 16.0705) (11.7401, 16.1136) knots 0 0 0 0 0.027067 0.049766 0.049766 0.049766 0.049766
  spline S132 degree 3 poles (11.7401, 16.1136) (11.6925, 16.1668) (11.5963, 16.2748) (11.5835, 16.419) (11.5771, 16.4921) knots 0 0 0 0 0.020829 0.042207 0.042207 0.042207 0.042207
  spline S133 degree 3 poles (11.5771, 16.4921) (11.5795, 16.5359) (11.5842, 16.6221) (11.6206, 16.7004) (11.6385, 16.739) knots 0 0 0 0 0.013021 0.025653 0.025653 0.025653 0.025653
  spline S134 degree 3 poles (11.6385, 16.739) (11.6604, 16.7742) (11.7034, 16.8437) (11.7679, 16.8937) (11.7996, 16.9184) knots 0 0 0 0 0.012324 0.024281 0.024281 0.024281 0.024281
  spline S135 degree 3 poles (11.7996, 16.9184) (11.8342, 16.9396) (11.9048, 16.983) (11.9838, 17.0079) (12.024, 17.0207) knots 0 0 0 0 0.01214 0.024739 0.024739 0.024739 0.024739
  spline S136 degree 3 poles (12.024, 17.0207) (12.0623, 17.0291) (12.1539, 17.0493) (12.247, 17.0608) (12.3012, 17.0675) knots 0 0 0 0 0.011765 0.028127 0.028127 0.028127 0.028127
  spline S137 degree 3 poles (12.3012, 17.0675) (12.4111, 17.0808) (12.5991, 17.1037) (12.7816, 17.1541) (12.8573, 17.1751) knots 0 0 0 0 0.033159 0.056713 0.056713 0.056713 0.056713
  spline S138 degree 3 poles (12.8573, 17.1751) (12.8578, 17.1925) (12.8585, 17.2197) (12.8589, 17.2468) (12.859, 17.2565) knots 0 0 0 0 0.005243 0.008145 0.008145 0.008145 0.008145
  spline S139 degree 3 poles (12.859, 17.2565) (12.8578, 17.3129) (12.8555, 17.4122) (12.7963, 17.491) (12.7706, 17.525) knots 0 0 0 0 0.016393 0.028904 0.028904 0.028904 0.028904
  spline S140 degree 3 poles (12.7706, 17.525) (12.7224, 17.5558) (12.6147, 17.6245) (12.4864, 17.6284) (12.4154, 17.6306) knots 0 0 0 0 0.01684 0.037669 0.037669 0.037669 0.037669
  spline S141 degree 3 poles (12.4154, 17.6306) (12.3502, 17.6296) (12.2357, 17.6278) (12.1343, 17.5758) (12.0905, 17.5534) knots 0 0 0 0 0.01922 0.03378 0.03378 0.03378 0.03378
  spline S142 degree 3 poles (12.0905, 17.5534) (12.0572, 17.5196) (11.9815, 17.443) (11.952, 17.3388) (11.9355, 17.2805) knots 0 0 0 0 0.014041 0.031838 0.031838 0.031838 0.031838
  line L99 (11.9355, 17.2805) -> (11.6306, 17.322)
  spline S143 degree 3 poles (11.6306, 17.322) (11.6455, 17.3825) (11.6733, 17.4958) (11.7375, 17.593) (11.7674, 17.6383) knots 0 0 0 0 0.01853 0.034683 0.034683 0.034683 0.034683
  spline S144 degree 3 poles (11.7674, 17.6383) (11.8043, 17.6766) (11.8826, 17.7582) (11.9874, 17.801) (12.0428, 17.8237) knots 0 0 0 0 0.01579 0.033533 0.033533 0.033533 0.033533
  spline S145 degree 3 poles (12.0428, 17.8237) (12.1072, 17.8427) (12.2434, 17.8828) (12.3855, 17.8867) (12.4604, 17.8888) knots 0 0 0 0 0.02005 0.042416 0.042416 0.042416 0.042416
  spline S146 degree 3 poles (12.4604, 17.8888) (12.5321, 17.8876) (12.6622, 17.8855) (12.7872, 17.8496) (12.8433, 17.8335) knots 0 0 0 0 0.021399 0.038838 0.038838 0.038838 0.038838
  spline S147 degree 3 poles (12.8433, 17.8335) (12.8877, 17.8154) (12.9689, 17.7824) (13.0316, 17.7216) (13.0599, 17.694) knots 0 0 0 0 0.014228 0.025974 0.025974 0.025974 0.025974
  spline S148 degree 3 poles (13.0599, 17.694) (13.0815, 17.6632) (13.1268, 17.5985) (13.1466, 17.522) (13.157, 17.4818) knots 0 0 0 0 0.011185 0.023506 0.023506 0.023506 0.023506
  spline S149 degree 3 poles (13.157, 17.4818) (13.1615, 17.4446) (13.173, 17.3491) (13.1728, 17.2529) (13.1726, 17.1942) knots 0 0 0 0 0.011236 0.028827 0.028827 0.028827 0.028827
  line L100 (13.1726, 17.1942) -> (13.1727, 16.7784)
  spline S150 degree 3 poles (13.1727, 16.7784) (13.1721, 16.6599) (13.171, 16.4762) (13.1871, 16.2933) (13.1928, 16.2283) knots 0 0 0 0 0.0355 0.055071 0.055071 0.055071 0.055071
  spline S151 degree 3 poles (13.1928, 16.2283) (13.2012, 16.1901) (13.218, 16.1131) (13.2537, 16.0428) (13.2717, 16.0074) knots 0 0 0 0 0.011667 0.02354 0.02354 0.02354 0.02354
  spline S152 degree 3 poles (9.5388, 16.0489) (9.477, 16.0365) (9.3418, 16.0095) (9.2039, 16.0075) (9.129, 16.0064) knots 0 0 0 0 0.018874 0.041272 0.041272 0.041272 0.041272
  line L101 (9.129, 16.0064) -> (8.1605, 16.0061)
  line L102 (8.1605, 16.0061) -> (8.1599, 18.5461)
  line L103 (8.1599, 18.5461) -> (9.1128, 18.5463)
  spline S153 degree 3 poles (9.1128, 18.5463) (9.2011, 18.5448) (9.3607, 18.5419) (9.5121, 18.4918) (9.5798, 18.4694) knots 0 0 0 0 0.026298 0.047566 0.047566 0.047566 0.047566
  spline S154 degree 3 poles (9.5798, 18.4694) (9.6351, 18.4403) (9.7454, 18.3826) (9.8188, 18.2821) (9.8553, 18.2321) knots 0 0 0 0 0.018485 0.036799 0.036799 0.036799 0.036799
  spline S155 degree 3 poles (9.8553, 18.2321) (9.8844, 18.1786) (9.9414, 18.0739) (9.9505, 17.9551) (9.955, 17.8968) knots 0 0 0 0 0.018017 0.035328 0.035328 0.035328 0.035328
  spline S156 degree 3 poles (9.955, 17.8968) (9.9512, 17.8431) (9.9435, 17.7347) (9.8925, 17.6386) (9.8667, 17.5901) knots 0 0 0 0 0.015964 0.032232 0.032232 0.032232 0.032232
  spline S157 degree 3 poles (9.8667, 17.5901) (9.8323, 17.5439) (9.7604, 17.4473) (9.655, 17.3885) (9.6, 17.3579) knots 0 0 0 0 0.017083 0.035728 0.035728 0.035728 0.035728
  spline S158 degree 3 poles (9.6, 17.3579) (9.6714, 17.3327) (9.8083, 17.2843) (9.9071, 17.1783) (9.9543, 17.1276) knots 0 0 0 0 0.022335 0.042827 0.042827 0.042827 0.042827
  spline S159 degree 3 poles (9.9543, 17.1276) (9.9905, 17.0701) (10.0644, 16.9525) (10.0736, 16.8138) (10.0783, 16.7429) knots 0 0 0 0 0.020043 0.040978 0.040978 0.040978 0.040978
  spline S160 degree 3 poles (10.0783, 16.7429) (10.0753, 16.6848) (10.0694, 16.5698) (10.025, 16.4636) (10.003, 16.4111) knots 0 0 0 0 0.017321 0.034254 0.034254 0.034254 0.034254
  spline S161 degree 3 poles (10.003, 16.4111) (9.9776, 16.3638) (9.9292, 16.274) (9.8529, 16.2065) (9.8168, 16.1746) knots 0 0 0 0 0.01598 0.030315 0.030315 0.030315 0.030315
  spline S162 degree 3 poles (9.8168, 16.1746) (9.7761, 16.1482) (9.6899, 16.0923) (9.591, 16.0639) (9.5388, 16.0489) knots 0 0 0 0 0.014472 0.030663 0.030663 0.030663 0.030663
  line L104 (2.8678, 14.591) -> (3.0687, 14.591)
  line L105 (3.0687, 14.591) -> (3.0694, 12.0406)
  line L106 (3.0694, 12.0406) -> (2.7575, 12.0405)
  line L107 (2.7575, 12.0405) -> (2.757, 14.0278)
  spline S163 degree 3 poles (2.757, 14.0278) (2.7145, 13.9908) (2.6224, 13.9106) (2.5179, 13.8471) (2.4617, 13.8129) knots 0 0 0 0 0.016876 0.036586 0.036586 0.036586 0.036586
  spline S164 degree 3 poles (2.4617, 13.8129) (2.4045, 13.7802) (2.2985, 13.7194) (2.1855, 13.6731) (2.1334, 13.6517) knots 0 0 0 0 0.01973 0.036608 0.036608 0.036608 0.036608
  line L108 (2.1334, 13.6517) -> (2.1333, 13.9532)
  spline S165 degree 3 poles (2.1333, 13.9532) (2.2169, 13.9956) (2.3802, 14.0785) (2.5216, 14.1947) (2.5906, 14.2513) knots 0 0 0 0 0.028036 0.054737 0.054737 0.054737 0.054737
  spline S166 degree 3 poles (2.5906, 14.2513) (2.6495, 14.3062) (2.7576, 14.4069) (2.8333, 14.5334) (2.8678, 14.591) knots 0 0 0 0 0.024016 0.04403 0.04403 0.04403 0.04403
  line L109 (1.54, 17.0094) -> (1.5402, 16.0044)
  line L110 (1.5402, 16.0044) -> (1.2284, 16.0044)
  line L111 (1.2284, 16.0044) -> (1.2279, 17.8444)
  line L112 (1.2279, 17.8444) -> (1.5086, 17.8445)
  line L113 (1.5086, 17.8445) -> (1.5086, 17.5828)
  spline S167 degree 3 poles (1.5086, 17.5828) (1.5846, 17.6713) (1.7388, 17.8508) (1.9746, 17.8743) (2.0942, 17.8862) knots 0 0 0 0 0.03363 0.068256 0.068256 0.068256 0.068256
  spline S168 degree 3 poles (2.0942, 17.8862) (2.1479, 17.884) (2.2529, 17.8796) (2.3518, 17.8439) (2.4, 17.8265) knots 0 0 0 0 0.016031 0.031322 0.031322 0.031322 0.031322
  spline S169 degree 3 poles (2.4, 17.8265) (2.4427, 17.8062) (2.5231, 17.768) (2.5815, 17.7011) (2.6088, 17.6697) knots 0 0 0 0 0.014014 0.026358 0.026358 0.026358 0.026358
  spline S170 degree 3 poles (2.6088, 17.6697) (2.6303, 17.6352) (2.6749, 17.5636) (2.6953, 17.4817) (2.7059, 17.4393) knots 0 0 0 0 0.012138 0.02514 0.02514 0.02514 0.02514
  spline S171 degree 3 poles (2.7059, 17.4393) (2.7109, 17.3997) (2.7236, 17.2991) (2.7234, 17.1976) (2.7233, 17.1361) knots 0 0 0 0 0.011982 0.030396 0.030396 0.030396 0.030396
  line L114 (2.7233, 17.1361) -> (2.7236, 16.0047)
  line L115 (2.7236, 16.0047) -> (2.4117, 16.0047)
  line L116 (2.4117, 16.0047) -> (2.4114, 17.1239)
  spline S172 degree 3 poles (2.4114, 17.1239) (2.4111, 17.1798) (2.4106, 17.2765) (2.3855, 17.3697) (2.375, 17.4089) knots 0 0 0 0 0.01668 0.028836 0.028836 0.028836 0.028836
  spline S173 degree 3 poles (2.375, 17.4089) (2.3602, 17.439) (2.3301, 17.5002) (2.2743, 17.5396) (2.2459, 17.5596) knots 0 0 0 0 0.009876 0.02013 0.02013 0.02013 0.02013
  spline S174 degree 3 poles (2.2459, 17.5596) (2.2129, 17.576) (2.1445, 17.6101) (2.068, 17.6139) (2.0284, 17.6159) knots 0 0 0 0 0.01092 0.022678 0.022678 0.022678 0.022678
  spline S175 degree 3 poles (2.0284, 17.6159) (1.9645, 17.6108) (1.838, 17.6008) (1.7353, 17.5262) (1.6845, 17.4893) knots 0 0 0 0 0.018828 0.037284 0.037284 0.037284 0.037284
  spline S176 degree 3 poles (1.6845, 17.4893) (1.6426, 17.4302) (1.5419, 17.2881) (1.5407, 17.1121) (1.54, 17.0094) knots 0 0 0 0 0.021294 0.051185 0.051185 0.051185 0.051185
  spline S177 degree 3 poles (-1.2935, 16.2931) (-1.2786, 16.2865) (-1.2448, 16.2717) (-1.2077, 16.271) (-1.187, 16.2706) knots 0 0 0 0 0.004831 0.010986 0.010986 0.010986 0.010986
  spline S178 degree 3 poles (-1.187, 16.2706) (-1.1669, 16.2713) (-1.121, 16.2729) (-1.0756, 16.2792) (-1.0501, 16.2827) knots 0 0 0 0 0.006029 0.013749 0.013749 0.013749 0.013749
  line L117 (-1.0501, 16.2827) -> (-1.005, 16.0073)
  spline S179 degree 3 poles (-1.005, 16.0073) (-1.0464, 15.9992) (-1.1243, 15.984) (-1.2035, 15.9809) (-1.2406, 15.9795) knots 0 0 0 0 0.012647 0.023757 0.023757 0.023757 0.023757
  spline S180 degree 3 poles (-1.2406, 15.9795) (-1.2916, 15.9805) (-1.3829, 15.9822) (-1.4669, 16.0175) (-1.504, 16.0331) knots 0 0 0 0 0.015133 0.027094 0.027094 0.027094 0.027094
  spline S181 degree 3 poles (-1.504, 16.0331) (-1.5326, 16.0519) (-1.5881, 16.0883) (-1.6202, 16.1463) (-1.6357, 16.1743) knots 0 0 0 0 0.010107 0.019568 0.019568 0.019568 0.019568
  spline S182 degree 3 poles (-1.6357, 16.1743) (-1.6466, 16.2194) (-1.676, 16.34) (-1.6747, 16.4645) (-1.6739, 16.5425) knots 0 0 0 0 0.013877 0.037135 0.037135 0.037135 0.037135
  line L118 (-1.6739, 16.5425) -> (-1.6742, 17.6011)
  line L119 (-1.6742, 17.6011) -> (-1.9029, 17.601)
  line L120 (-1.9029, 17.601) -> (-1.9029, 17.8436)
  line L121 (-1.9029, 17.8436) -> (-1.6742, 17.8437)
  line L122 (-1.6742, 17.8437) -> (-1.6743, 18.2993)
  line L123 (-1.6743, 18.2993) -> (-1.3642, 18.4865)
  line L124 (-1.3642, 18.4865) -> (-1.3641, 17.8437)
  line L125 (-1.3641, 17.8437) -> (-1.0505, 17.8438)
  line L126 (-1.0505, 17.8438) -> (-1.0504, 17.6013)
  line L127 (-1.0504, 17.6013) -> (-1.364, 17.6012)
  line L128 (-1.364, 17.6012) -> (-1.3638, 16.5252)
  spline S183 degree 3 poles (-1.3638, 16.5252) (-1.3642, 16.4885) (-1.3649, 16.4306) (-1.352, 16.3743) (-1.3472, 16.3537) knots 0 0 0 0 0.010966 0.017282 0.017282 0.017282 0.017282
  spline S184 degree 3 poles (-1.3472, 16.3537) (-1.3408, 16.3416) (-1.3278, 16.3171) (-1.305, 16.3011) (-1.2935, 16.2931) knots 0 0 0 0 0.00405 0.008204 0.008204 0.008204 0.008204
  line L129 (-5.6745, 16.7719) -> (-5.9533, 16.0026)
  line L130 (-5.9533, 16.0026) -> (-6.3102, 16.0025)
  line L131 (-6.3102, 16.0025) -> (-5.3354, 18.5427)
  line L132 (-5.3354, 18.5427) -> (-4.9733, 18.5428)
  line L133 (-4.9733, 18.5428) -> (-3.9331, 16.0031)
  line L134 (-3.9331, 16.0031) -> (-4.316, 16.003)
  line L135 (-4.316, 16.003) -> (-4.6124, 16.7722)
  line L136 (-4.6124, 16.7722) -> (-5.6745, 16.7719)
  spline S185 degree 3 poles (-9.3831, 16.291) (-9.3682, 16.2845) (-9.3343, 16.2696) (-9.2973, 16.2689) (-9.2765, 16.2685) knots 0 0 0 0 0.004831 0.010986 0.010986 0.010986 0.010986
  spline S186 degree 3 poles (-9.2765, 16.2685) (-9.2564, 16.2693) (-9.2106, 16.2709) (-9.1651, 16.2772) (-9.1396, 16.2807) knots 0 0 0 0 0.006028 0.013749 0.013749 0.013749 0.013749
  line L137 (-9.1396, 16.2807) -> (-9.0945, 16.0052)
  spline S187 degree 3 poles (-9.0945, 16.0052) (-9.136, 15.9971) (-9.2138, 15.982) (-9.2931, 15.9789) (-9.3301, 15.9775) knots 0 0 0 0 0.012647 0.023757 0.023757 0.023757 0.023757
  spline S188 degree 3 poles (-9.3301, 15.9775) (-9.3811, 15.9784) (-9.4725, 15.9802) (-9.5564, 16.0155) (-9.5935, 16.0311) knots 0 0 0 0 0.015133 0.027094 0.027094 0.027094 0.027094
  spline S189 degree 3 poles (-9.5935, 16.0311) (-9.6222, 16.0499) (-9.6776, 16.0863) (-9.7097, 16.1442) (-9.7252, 16.1723) knots 0 0 0 0 0.010107 0.019568 0.019568 0.019568 0.019568
  spline S190 degree 3 poles (-9.7252, 16.1723) (-9.7362, 16.2174) (-9.7655, 16.338) (-9.7642, 16.4625) (-9.7634, 16.5404) knots 0 0 0 0 0.013877 0.037135 0.037135 0.037135 0.037135
  line L138 (-9.7634, 16.5404) -> (-9.7637, 17.5991)
  line L139 (-9.7637, 17.5991) -> (-9.9924, 17.599)
  line L140 (-9.9924, 17.599) -> (-9.9925, 17.8416)
  line L141 (-9.9925, 17.8416) -> (-9.7638, 17.8416)
  line L142 (-9.7638, 17.8416) -> (-9.7639, 18.2973)
  line L143 (-9.7639, 18.2973) -> (-9.4538, 18.4845)
  line L144 (-9.4538, 18.4845) -> (-9.4536, 17.8417)
  line L145 (-9.4536, 17.8417) -> (-9.14, 17.8418)
  line L146 (-9.14, 17.8418) -> (-9.14, 17.5992)
  line L147 (-9.14, 17.5992) -> (-9.4536, 17.5991)
  line L148 (-9.4536, 17.5991) -> (-9.4533, 16.5232)
  spline S191 degree 3 poles (-9.4533, 16.5232) (-9.4537, 16.4864) (-9.4544, 16.4285) (-9.4415, 16.3722) (-9.4368, 16.3517) knots 0 0 0 0 0.010966 0.017282 0.017282 0.017282 0.017282
  spline S192 degree 3 poles (-9.4368, 16.3517) (-9.4303, 16.3396) (-9.4173, 16.3151) (-9.3946, 16.2991) (-9.3831, 16.291) knots 0 0 0 0 0.00405 0.008204 0.008204 0.008204 0.008204
  spline S193 degree 3 poles (-13.0206, 15.9592) (-13.1418, 15.9681) (-13.3765, 15.9852) (-13.5576, 16.1346) (-13.6452, 16.2068) knots 0 0 0 0 0.035479 0.06869 0.06869 0.06869 0.06869
  spline S194 degree 3 poles (-13.6452, 16.2068) (-13.7146, 16.3041) (-13.8661, 16.5166) (-13.8775, 16.7786) (-13.8837, 16.9206) knots 0 0 0 0 0.035119 0.076697 0.076697 0.076697 0.076697
  spline S195 degree 3 poles (-13.8837, 16.9206) (-13.8766, 17.0755) (-13.8636, 17.3603) (-13.6824, 17.5783) (-13.5997, 17.6778) knots 0 0 0 0 0.045048 0.082857 0.082857 0.082857 0.082857
  spline S196 degree 3 poles (-13.5997, 17.6778) (-13.515, 17.7374) (-13.3414, 17.8596) (-13.1295, 17.8747) (-13.0211, 17.8824) knots 0 0 0 0 0.030474 0.062419 0.062419 0.062419 0.062419
  spline S197 degree 3 poles (-13.0211, 17.8824) (-12.9015, 17.8732) (-12.6683, 17.8552) (-12.4884, 17.7064) (-12.4007, 17.6339) knots 0 0 0 0 0.035035 0.068301 0.068301 0.068301 0.068301
  spline S198 degree 3 poles (-12.4007, 17.6339) (-12.3305, 17.5389) (-12.1803, 17.3355) (-12.1669, 17.082) (-12.1597, 16.947) knots 0 0 0 0 0.034681 0.074234 0.074234 0.074234 0.074234
  spline S199 degree 3 poles (-12.1597, 16.947) (-12.1618, 16.8398) (-12.1655, 16.6471) (-12.2352, 16.4678) (-12.2661, 16.3882) knots 0 0 0 0 0.03184 0.057276 0.057276 0.057276 0.057276
  spline S200 degree 3 poles (-12.2661, 16.3882) (-12.3058, 16.3241) (-12.3854, 16.1954) (-12.5124, 16.1132) (-12.5762, 16.0719) knots 0 0 0 0 0.022319 0.044787 0.044787 0.044787 0.044787
  spline S201 degree 3 poles (-12.5762, 16.0719) (-12.646, 16.0391) (-12.7868, 15.9727) (-12.9422, 15.9637) (-13.0206, 15.9592) knots 0 0 0 0 0.022904 0.046226 0.046226 0.046226 0.046226
  spline S202 degree 3 poles (-16.7405, 16.2147) (-16.6862, 16.2179) (-16.5811, 16.2242) (-16.4912, 16.2786) (-16.4478, 16.3049) knots 0 0 0 0 0.016055 0.031049 0.031049 0.031049 0.031049